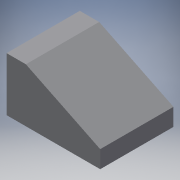
# Autodesk Inventor part: Work Planes
Saved by Autodesk Inventor 2016 (Build 200138000, 138)
## iProperties
Created: 2013-12-03
Part Number: Work Planes
Material: Generic
Document SubType Name: Modeling
Designer: John
Density: 1 g/cm^3
Appearance: Default
Author: John
Autodesk Inventor part; units mm, degrees
ref_plane "YZ Plane" through (0, 0, 0) normal (1, 0, 0) x (0, 1, 0)
ref_plane "XZ Plane" through (0, 0, 0) normal (0, 1, 0) x (-1, 0, 0)
ref_plane "XY Plane" through (0, 0, 0) normal (0, 0, 1) x (1, 0, 0)
sketch "Sketch1" plane through (0, 0, 0) normal (0, 0, 1) x (1, 0, 0)
  line L0 (0, 0) -> (32.4623, 0)
  line L1 (32.4623, 0) -> (32.4623, 18.6079)
  line L2 (32.4623, 18.6079) -> (0, 18.6079)
  line L3 (0, 18.6079) -> (0, 0)
  constraints: 8 end point, 2 parallel, 1 horizontal, 1 perpendicular
extrude "Extrusion1" add sketch "Sketch1" along normal blind 25.4
sketch "Sketch2" plane through (0, 0, 25.4) normal (0, 0, 1) x (1, 0, 0)
  line L0 (32.4623, 0) -> (32.4623, 18.6079) projected
  line L1 (32.4623, 18.6079) -> (0, 18.6079) projected
  line L2 (6.7125, 18.6079) -> (32.4623, 6.0135)
  constraints: 2 end point, 2 point on line
extrude "Extrusion2" cut sketch "Sketch2" against normal through all
body "Solid1"
